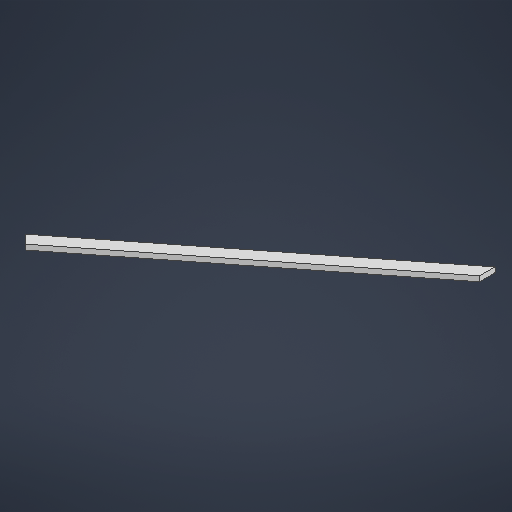
# Autodesk Inventor part: S_2x4x96.546
Saved by Autodesk Inventor 2026 (Build 300175000, 175)
## iProperties
Created: 2025-09-08
Part Number: S_2x4x96.546
Material: Generic
Document SubType Name: Modeling
Designer: trott
Density: 1 g/cm^3
Appearance: Default
Author: trott
Autodesk Inventor part; units mm, degrees
ref_plane "YZ Plane" through (0, 0, 0) normal (1, 0, 0) x (0, 1, 0)
ref_plane "XZ Plane" through (0, 0, 0) normal (0, 1, 0) x (-1, 0, 0)
ref_plane "XY Plane" through (0, 0, 0) normal (0, 0, 1) x (1, 0, 0)
sketch "Sketch1" plane through (0, 0, 0) normal (0, 1, 0) x (-1, 0, 0)
  line L0 (0, 0) -> (0, -1219.2)
  line L1 (0, 0) -> (88.9, 0)
  line L2 (88.9, 0) -> (88.9, -1219.2)
  line L3 (88.9, -1219.2) -> (0, -1219.2)
  line L4 (0, 0) -> (0, 1219.2) construction
  line L5 (0, 1219.2) -> (1219.2, 1219.2) construction
  line L6 (0, 1219.2) -> (0, 3657.6) construction
  line L7 (0, 3657.6) -> (0, 4876.8) construction
  line L8 (0, 4876.8) -> (0, 6096) construction
  line L9 (0, -1219.2) -> (2438.4, -1219.2) construction
  line L10 (0, 6096) -> (2438.4, 6096) construction
  line L11 (2438.4, 6096) -> (2438.4, -1219.2) construction
  line L12 (0, 3657.6) -> (0, 3352.8) construction
  line L13 (0, 3352.8) -> (2438.4, 3352.8) construction
  line L14 (2438.4, 3352.8) -> (1219.2, 3352.8)
  line L15 (1219.2, 3352.8) -> (1219.2, 3263.9)
  line L16 (1219.2, 3263.9) -> (2438.4, 3263.9)
  line L17 (2438.4, 3263.9) -> (2438.4, 3352.8)
  line L18 (0, 6096) -> (862.1046, 6958.1046)
  line L19 (862.1046, 6958.1046) -> (924.9664, 6895.2428)
  line L20 (924.9664, 6895.2428) -> (62.8618, 6033.1382)
  line L21 (62.8618, 6033.1382) -> (0, 6096)
  line L22 (0, 4876.8) -> (1219.2, 4876.8) construction
  line L23 (1219.2, 4876.8) -> (2081.3046, 5738.9046)
  line L24 (1219.2, 1219.2) -> (2081.3046, 357.0954)
  line L25 (2081.3046, 357.0954) -> (2018.4428, 294.2336)
  line L26 (2018.4428, 294.2336) -> (1156.3382, 1156.3382)
  line L27 (1156.3382, 1156.3382) -> (1219.2, 1219.2)
  line L28 (2018.4428, 294.2336) -> (88.9, -1219.2)
  line L29 (2081.3046, 357.0954) -> (2144.1664, 419.9572)
  line L30 (2144.1664, 419.9572) -> (1282.0618, 1282.0618)
  line L31 (1282.0618, 1282.0618) -> (1219.2, 1219.2)
  line L32 (2438.4, 3352.8) -> (2438.4, 3441.7)
  line L33 (2438.4, 3441.7) -> (1219.2, 3441.7)
  line L34 (1219.2, 3441.7) -> (1219.2, 3352.8)
  line L35 (1156.3382, 4939.6618) -> (1282.0618, 4813.9382)
  line L36 (2018.4428, 5801.7664) -> (2144.1664, 5676.0428)
  line L37 (1282.0618, 4813.9382) -> (2144.1664, 5676.0428)
  line L38 (2018.4428, 5801.7664) -> (1156.3382, 4939.6618)
  line L39 (2018.4428, 5801.7664) -> (924.9664, 6895.2428)
  line L40 (62.8618, 6033.1382) -> (1156.3382, 4939.6618)
  line L41 (1233.6206, 4168.8855) -> (1267.6412, 4086.7527)
  line L42 (1263.7078, 2313.9849) -> (1230.0006, 2231.7229)
  arc A0 (862.1046, 6958.1046) -> (0, 6096) centre (431.0523, 6527.0523) ccw
  line L43 (1246.8542, 2272.8539) -> (2375.0183, 1810.583)
  line L44 (2391.8719, 1851.7139) -> (2358.1646, 1769.452)
  line L45 (2391.8719, 1851.7139) -> (1263.7078, 2313.9849)
  line L46 (1230.0006, 2231.7229) -> (2358.1646, 1769.452)
  line L47 (1282.0618, 1282.0618) -> (1230.0006, 2231.7229)
  line L48 (1230.0006, 2231.7229) -> (1219.2, 3263.9)
  line L49 (2144.1664, 419.9572) -> (2391.8719, 1851.7139)
  line L50 (2391.8719, 1851.7139) -> (2438.4, 3263.9)
  line L51 (1219.2, 3441.7) -> (1233.6206, 4168.8855)
  line L52 (1233.6206, 4168.8855) -> (1282.0618, 4813.9382)
  line L53 (1250.6309, 4127.8191) -> (2377.0248, 4594.3867)
  line L54 (2360.0145, 4635.4532) -> (2394.0351, 4553.3203)
  line L55 (2394.0351, 4553.3203) -> (1267.6412, 4086.7527)
  line L56 (2360.0145, 4635.4532) -> (1233.6206, 4168.8855)
  line L57 (2394.0351, 4553.3203) -> (2144.1664, 5676.0428)
  line L58 (2438.4, 3441.7) -> (2394.0351, 4553.3203)
  line L59 (2144.1664, 5676.0428) -> (2057.3895, 5656.7301)
  line L60 (2394.0351, 4553.3203) -> (2305.2058, 4549.7751)
  line L61 (2394.0351, 4553.3203) -> (2307.2582, 4534.0076)
  line L62 (2307.2582, 4534.0076) -> (2057.3895, 5656.7301)
  line L63 (2438.4, 3441.7) -> (2349.5707, 3438.1548)
  line L64 (2349.5707, 3438.1548) -> (2305.2058, 4549.7751)
  line L65 (1219.2, 3441.7) -> (1308.0825, 3439.9374)
  line L66 (1233.6206, 4168.8855) -> (1322.5031, 4167.1229)
  line L67 (1322.5031, 4167.1229) -> (1308.0825, 3439.9374)
  line L68 (1282.0618, 4813.9382) -> (1292.2698, 4949.8698)
  line L69 (1292.2698, 4949.8698) -> (1380.9202, 4943.2124)
  line L70 (1233.6206, 4168.8855) -> (1322.271, 4162.2282)
  line L71 (1322.271, 4162.2282) -> (1380.9202, 4943.2124)
  line L72 (2018.4428, 5801.7664) -> (1955.581, 5738.9046)
  line L73 (1955.581, 5738.9046) -> (862.1046, 6832.381)
  line L74 (924.9664, 6895.2428) -> (862.1046, 6832.381)
  line L75 (62.8618, 6033.1382) -> (125.7236, 6096)
  line L76 (62.8618, 6033.1382) -> (125.7236, 6096)
  line L77 (125.7236, 6096) -> (1219.2, 5002.5236)
  line L78 (1156.3382, 1156.3382) -> (0, 0)
  line L79 (0, 0) -> (62.8618, -62.8618)
  line L80 (1156.3382, 1156.3382) -> (1219.2, 1093.4764)
  line L81 (1219.2, 1093.4764) -> (62.8618, -62.8618)
  line L82 (2018.4428, 294.2336) -> (1963.5776, 364.1837)
  line L83 (88.9, -1219.2) -> (34.0348, -1149.2499)
  line L84 (34.0348, -1149.2499) -> (1963.5776, 364.1837)
  line L85 (2144.1664, 419.9572) -> (2056.5677, 435.1125)
  line L86 (2391.8719, 1851.7139) -> (2304.2732, 1866.8692)
  line L87 (2391.8719, 1851.7139) -> (2303.0201, 1854.6414)
  line L88 (2304.2732, 1866.8692) -> (2056.5677, 435.1125)
  line L89 (1282.0618, 1282.0618) -> (1289.3538, 1149.0462)
  line L90 (1289.3538, 1149.0462) -> (1378.1205, 1153.9124)
  line L91 (1230.0006, 2231.7229) -> (1318.7673, 2236.5892)
  line L92 (1230.0006, 2231.7229) -> (1318.8957, 2232.6531)
  line L93 (1318.7673, 2236.5892) -> (1378.1205, 1153.9124)
  line L94 (1219.2, 3263.9) -> (1308.0951, 3264.8302)
  line L95 (1308.0951, 3264.8302) -> (1318.8957, 2232.6531)
  line L96 (2438.4, 3263.9) -> (2349.5482, 3266.8275)
  line L97 (2349.5482, 3266.8275) -> (2303.0201, 1854.6414)
  point P0 (1770.957, 2057.4547)
  point P1 (1955.1236, 357.5528)
  point P2 (88.9, -1106.2164)
  dimension "d0" = 1219.2
  dimension "d2" = 1219.2
  dimension "d3" = 1219.2
  dimension "d16" = 2438.4
  dimension "d17" = 1219.2
  dimension "d18" = 1219.2
  dimension "d20" = 2438.4
  dimension "d21" = 304.8
  dimension "d22" = 1219.2
  dimension "d23" = 88.9
  dimension "d24" = 1219.2
  dimension "d25" = 45
  dimension "d26" = 88.9
  dimension "d27" = 1219.2
  dimension "d28" = 1219.2
  dimension "d29" = 1219.2
  dimension "d31" = 1219.2
  dimension "d32" = 88.9
  dimension "d33" = 88.9
  dimension "d34" = 88.9
  dimension "d35" = 177.8
  dimension "d36" = 177.8
  dimension "d38" = 88.9
  dimension "d39" = 88.9
  dimension "d43" = 1219.2
  dimension "d44" = 88.9
  dimension "d45" = 1219.2
  dimension "d46" = 88.9
  dimension "d47" = 88.9
  dimension "d48" = 88.9
  dimension "d49" = 88.9
  dimension "d50" = 88.9
  dimension "d51" = 88.9
  dimension "d52" = 88.9
  dimension "d53" = 88.9
  dimension "d54" = 88.9
  dimension "d55" = 88.9
  dimension "d57" = 88.9
  dimension "d58" = 88.9
  dimension "d59" = 88.9
  dimension "d60" = 88.9
  dimension "d61" = 88.9
  dimension "d62" = 88.9
  dimension "d63" = 88.9
  dimension "d64" = 88.9
  dimension "d65" = 88.9
  dimension "d66" = 88.9
  constraints: 196 end point, 42 perpendicular, 13 point on line, 8 midpoint, 5 horizontal, 4 parallel, 2 collinear, 2 point on circle, 2 vertical, 1 centre point
  measures "d0" distance of L0.start L0.end
  measures "d2" distance of L0.start L4.end
  measures "d3" distance of L4.end L5.end
  measures "d16" distance of L4.end L6.end
  measures "d17" distance of L6.end L7.end
  measures "d18" distance of L8.end L7.end
  measures "d20" distance of L8.end L10.end
  measures "d21" distance of L6.end L12.end
  measures "d22" distance of L13.end L14.end
  measures "d23" distance of L14.end L15.end
  measures "d24" distance of L8.end L18.end
  measures "d25" angle of L10 L18
  measures "d26" distance of L18.end L19.end
  measures "d27" distance of L19.end L20.end
  measures "d28" distance of L7.end L22.end
  measures "d29" distance of L22.end L23.end
  measures "d31" distance of L5.end L24.end
  measures "d32" distance of L24.end L25.end
  measures "d33" distance of L24.end L29.end
  measures "d34" distance of L13.end L32.end
  measures "d35" distance of L35.start L35.end
  measures "d36" distance of L36.start L36.end
  measures "d38" distance of L41.start L41.end
  measures "d39" distance of L42.start L42.end
  measures "d43" distance of L43.start L43.end
  measures "d44" distance of L44.start L44.end
  measures "d45" distance of L53.start L53.end
  measures "d46" distance of L36.end L59.end
  measures "d47" distance of L54.end L60.end
  measures "d48" distance of L54.end L61.end
  measures "d49" distance of L32.end L63.end
  measures "d50" distance of L33.end L65.end
  measures "d51" distance of L41.start L66.end
  measures "d52" distance of L68.end L69.end
  measures "d53" distance of L41.start L70.end
  measures "d54" distance of L20.end L75.end
  measures "d55" distance of L26.end L80.end
  measures "d57" distance of L25.end L82.end
  measures "d58" distance of L2.end L83.end
  measures "d59" distance of L29.end L85.end
  measures "d60" distance of L44.start L86.end
  measures "d61" distance of L44.start L87.end
  measures "d62" distance of L89.end L90.end
  measures "d63" distance of L42.end L91.end
  measures "d64" distance of L42.end L92.end
  measures "d65" distance of L15.end L94.end
  measures "d66" distance of L16.end L96.end
extrude "Extrusion1" add sketch "Sketch1" along normal blind 38.1 contours L2 L84 L26 L28
body "Solid1"
